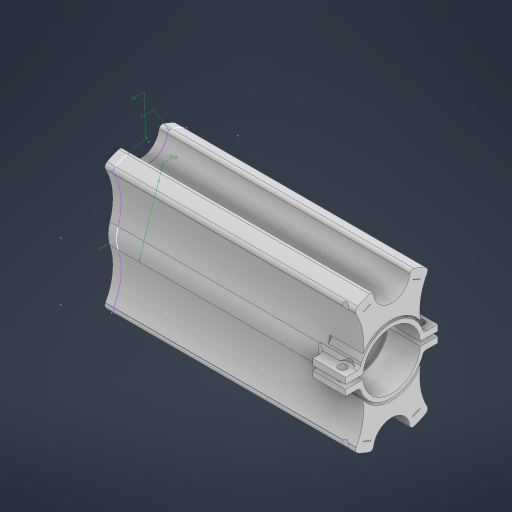
# Autodesk Inventor part: michigandrummy
Saved by Autodesk Inventor 2024.2 (Build 282272000, 272)
## iProperties
Created: 2024-04-03
Part Number: michigandrummy
Material: Generic
Document SubType Name: Modeling
Designer: jerem
Density: 1 g/cm^3
Appearance: Default
Author: jerem
## iProperties of the stored document michigandrummy_3DPrint.ipt
Created: 2024-04-05
Part Number: michigandrummy_3DPrint
Material: Generic
Document SubType Name: Modeling
Designer: jerem
Density: 1 g/cm^3
Appearance: Default
Author: jerem
Autodesk Inventor part; units mm, degrees
ref_plane "YZ Plane" through (0, 0, 0) normal (1, 0, 0) x (0, 1, 0)
ref_plane "XZ Plane" through (0, 0, 0) normal (0, 1, 0) x (-1, 0, 0)
ref_plane "XY Plane" through (0, 0, 0) normal (0, 0, 1) x (1, 0, 0)
sketch "Sketch1" plane through (0, 0, 0) normal (1, 0, 0) x (0, 1, 0)
  arc A0 (1, -13.863982) -> (1, 13.863982) centre (0, 0) ccw
  line L0 (0, 0) -> (1, 0) construction
  line L1 (1, 13.863982) -> (1, 22.388632)
  line L2 (1, 22.388632) -> (4, 22.388632)
  line L3 (4, 22.388632) -> (4, 15.388632)
  line L4 (1, -13.863982) -> (1, -22.388632)
  line L5 (1, -22.388632) -> (4, -22.388632)
  line L6 (4, -22.388632) -> (4, -15.388632)
  arc A1 (4, -15.388632) -> (4, 15.388632) centre (0, 0) ccw
  point P0 (4, -15.388632)
  point P1 (4, 15.388632)
  dimension "d0" = 27.8
  dimension "d1" = 1
  dimension "d3" = 3
  dimension "d4" = 2
  dimension "d5" = 1
  dimension "d11" = 7
  constraints: 14 end point, 4 point on circle, 2 centre point, 2 coincident, 2 collinear, 2 horizontal, 2 symmetric about line, 1 perpendicular, 1 vertical
  measures "d0" diameter of A0
  measures "d1" distance of L0.start L0.end
  measures "d3" distance of L1.end L2.end
  measures "d4" radial gap between concentric circles of A0 A1
  measures "d5" distance from line of point (0, 0) L1
  measures "d11" distance of L3.end L2.end
extrude "Extrusion1" add sketch "Sketch1" along normal blind 16
sketch "Sketch2" plane through (0, 4, 22.388632) normal (0, 1, 0) x (1, 0, 0)
  line L0 (0, 7) -> (16, 7) construction
  line L1 (16, 0) -> (16, 8.52465) construction
  line L2 (16, 7) -> (16, 0) construction
  circle A0 centre (11, 3.5) radius 2
  line L3 (16, 36.252614) -> (16, 8.52465)
  line L4 (16, 22.388632) -> (0, 22.388632)
  circle A1 centre (11, 41.277264) radius 2
  line L5 (11, 41.277264) -> (11, 37.777264) construction
  line L6 (0, 37.777264) -> (16, 37.777264) construction
  line L7 (11, 3.5) -> (11, 7) construction
  point P0 (16, 3.5)
  dimension "d8" = 5
  dimension "d9" = 4
  dimension "d10" = 3.5
  constraints: 8 end point, 3 point on line, 2 centre point, 2 midpoint, 1 collinear, 1 horizontal, 1 symmetric about line, 1 vertical, 1 other
  measures "d8" distance of point (16, 3.5) L7.start
  measures "d9" diameter of A0
  measures "d10" distance of L7.start L7.end
extrude "Extrusion2" cut sketch "Sketch2" along normal through all both and the other way through all
mirror "Mirror1" about plane through (0, 0, 0) normal (0, 1, 0) of "Extrusion1", "Extrusion2"
fillet "Fillet1" radius 2 4 edges at (8, 4, 15.3886) (8, -4, 15.3886) (8, 4, -15.3886) (8, -4, -15.3886)
sketch "Sketch3" plane through (0, -4, -22.388632) normal (-1, 0, 0) x (0, 0, 1)
  circle A0 centre (22.388632, 4) radius 13.9
  circle A1 centre (22.388632, 4) radius 15.9
  circle A2 centre (22.388632, 4) radius 4.85
  dimension "d15" = 9.7
  dimension "d19" = 27.8
  dimension "d20" = 2
  constraints: 3 centre point, 3 coincident
  measures "d15" diameter of A2
  measures "d19" diameter of A0
  measures "d20" radial gap between concentric circles of A0 A1
extrude "Extrusion3" add sketch "Sketch3" along normal blind 4.2 contours A0 | A1
sketch "Sketch4" plane through (-4.2, 0, 0) normal (-1, 0, 0) x (0, 0, 1)
  circle A0 centre (0, 0) radius 4.85 projected
  circle A1 centre (0, 0) radius 15.9
  circle A2 centre (0, 0) radius 4.85 projected
  circle A3 centre (0, 0) radius 1.8
  dimension "d18" = 3.6
  dimension "d21" = 31.8
  constraints: 2 centre point, 2 coincident
  measures "d18" diameter of A3
  measures "d21" diameter of A1
extrude "Extrusion4" add sketch "Sketch4" along normal blind 10 contours A0 | A1
fillet "Fillet2" radius 4 4 edges at (0, -3.1958, 15.5755) (0, 3.1958, 15.5755) (0, -3.1958, -15.5755) (0, 3.1958, -15.5755)
sketch "Sketch5" plane through (-14.2, 0, 0) normal (-1, 0, 0) x (0, 0, 1)
  circle A0 centre (0, 0) radius 1.8 projected
  circle A1 centre (0, 0) radius 2
  circle A2 centre (0, 0) radius 4
  dimension "d25" = 4
  dimension "d26" = 2
  constraints: 2 centre point, 2 coincident
  measures "d25" diameter of A1
  measures "d26" radial gap between concentric circles of A1 A2
extrude "Extrusion5" add sketch "Sketch5" along normal blind 87.8 contours A2
sketch "Sketch6" plane through (0, 0, 0) normal (1, 0, 0) x (0, 1, 0)
  circle A0 centre (0, 0) radius 1.8 construction
  circle A1 centre (0, 0) radius 35 construction
  line L0 (35, 0) -> (25, 0)
  line L1 (31.653557, -14.934936) -> (22.609684, -10.667811)
  arc A2 (31.653557, -14.934936) -> (35, 0) centre (0, 0) ccw construction
  dimension "d29" = 70
  dimension "d30" = 10
  dimension "d31" = 10
  constraints: 4 end point, 4 point on circle, 2 centre point, 1 coincident, 1 concentric, 1 horizontal, 1 line through centre
  measures "d29" diameter of A1
  measures "d30" distance of L0.start L0.end
  measures "d31" distance of L1.start L1.end
sketch "Sketch7" plane through (-102, 0, 0) normal (-1, 0, 0) x (0, 0, 1)
  circle A0 centre (0, 0) radius 15.9
  circle A1 centre (0, 0) radius 1.8
  line L0 (0, 0) -> (24.747716, 0) construction
  line L1 (-24.908169, 0) -> (-15.9, 0)
  line L2 (-1.8, 0) -> (15.9, 0)
  line L3 (17.349325, 28.247602) -> (17.271273, 28.112413)
  line L4 (0.160452, 0) -> (15.9, 0)
  arc A2 (0, 24.132295) -> (8.826003, 31.826928) centre (0, 33.041473) ccw
  arc A3 (17.349325, 28.247602) -> (15.118967, 4.922077) centre (43.063145, 14.019484) ccw
  arc A4 (0, 24.132295) -> (8.851951, 32.033302) centre (0, 33.041473) ccw
  arc A5 (16.480993, 30.876801) -> (10.805405, 33.290287) centre (0, 0) ccw
  line L5 (0, 15.9) -> (0, 24.132295)
  line L6 (-17.349325, 28.247602) -> (-17.271273, 28.112413)
  arc A6 (-15.118967, 4.922077) -> (-17.349325, 28.247602) centre (-43.063145, 14.019484) ccw
  arc A7 (-8.851951, 32.033302) -> (0, 24.132295) centre (0, 33.041473) ccw
  arc A8 (-10.805405, 33.290287) -> (-16.480993, 30.876801) centre (0, 0) ccw
  arc A9 (-16.480993, 30.876801) -> (-17.271273, 28.112413) centre (-15.539222, 29.112413) ccw
  arc A10 (17.271273, 28.112413) -> (16.480993, 30.876801) centre (15.539222, 29.112413) ccw
  arc A11 (-8.851951, 32.033302) -> (-10.805405, 33.290287) centre (-10.342316, 31.863561) ccw
  arc A12 (10.805405, 33.290287) -> (8.851951, 32.033302) centre (10.342316, 31.863561) ccw
  line L7 (17.349325, -28.247602) -> (17.271273, -28.112413)
  arc A13 (8.826003, -31.826928) -> (0, -24.132295) centre (0, -33.041473) ccw
  arc A14 (15.118967, -4.922077) -> (17.349325, -28.247602) centre (43.063145, -14.019484) ccw
  arc A15 (8.851951, -32.033302) -> (0, -24.132295) centre (0, -33.041473) ccw
  arc A16 (10.805405, -33.290287) -> (16.480993, -30.876801) centre (0, 0) ccw
  line L8 (0, -15.9) -> (0, -24.132295)
  arc A17 (-16.480993, -30.876801) -> (-10.805405, -33.290287) centre (0, 0) ccw
  arc A18 (-17.349325, -28.247602) -> (-15.118967, -4.922077) centre (-43.063145, -14.019484) ccw
  line L9 (-17.349325, -28.247602) -> (-17.271273, -28.112413)
  arc A19 (0, -24.132295) -> (-8.851951, -32.033302) centre (0, -33.041473) ccw
  arc A20 (-17.271273, -28.112413) -> (-16.480993, -30.876801) centre (-15.539222, -29.112413) ccw
  arc A21 (16.480993, -30.876801) -> (17.271273, -28.112413) centre (15.539222, -29.112413) ccw
  arc A22 (-10.805405, -33.290287) -> (-8.851951, -32.033302) centre (-10.342316, -31.863561) ccw
  arc A23 (8.851951, -32.033302) -> (10.805405, -33.290287) centre (10.342316, -31.863561) ccw
  point P0 (18.274622, 29.850263)
  point P1 (-8.826003, 31.826928)
  point P2 (-18.274622, 29.850263)
  point P3 (18.274622, -29.850263)
  point P4 (-8.826003, -31.826928)
  point P5 (-18.274622, -29.850263)
  point P6 (8.826003, 31.826928)
  point P7 (-15.118967, 4.922077)
  point P8 (-15.118967, -4.922077)
  point P9 (15.118967, -4.922077)
  dimension "d36" = 35
  dimension "d40" = 1.5
  dimension "d41" = 31.8
  constraints: 54 point on circle, 30 symmetric about line, 23 centre point, 20 end point, 9 tangent, 6 point on line, 4 coincident, 2 equal radius, 1 horizontal, 1 horizontal alignment, 15 other
  measures "d36" radius of A5
  measures "d40" radius of A11
  measures "d41" diameter of A0
extrude "Extrusion6" add sketch "Sketch7" against normal up to surface (87.8 mm away)
sketch "Sketch8" plane through (-14.2, 0, 0) normal (1, 0, 0) x (0, 0, -1)
  circle A0 centre (0, 0) radius 35
  circle A1 centre (0, 0) radius 15.9
  arc A2 (-17.349325, -28.247602) -> (-15.118967, -4.922077) centre (-43.063145, -14.019484) ccw
  arc A3 (15.118967, 4.922077) -> (-15.118967, 4.922077) centre (0, 0) ccw
  arc A4 (17.349325, 28.247602) -> (15.118967, 4.922077) centre (43.063145, 14.019484) ccw
  line L0 (17.349325, 28.247602) -> (17.271273, 28.112413)
  arc A5 (17.271273, 28.112413) -> (16.480993, 30.876801) centre (15.539222, 29.112413) ccw
  arc A6 (16.480993, 30.876801) -> (10.805405, 33.290287) centre (0, 0) ccw
  arc A7 (10.805405, 33.290287) -> (8.851951, 32.033302) centre (10.342316, 31.863561) ccw
  arc A8 (-8.851951, 32.033302) -> (8.851951, 32.033302) centre (0, 33.041473) ccw
  arc A9 (-8.851951, 32.033302) -> (-10.805405, 33.290287) centre (-10.342316, 31.863561) ccw
  arc A10 (-10.805405, 33.290287) -> (-16.480993, 30.876801) centre (0, 0) ccw
  arc A11 (-16.480993, 30.876801) -> (-17.271273, 28.112413) centre (-15.539222, 29.112413) ccw
  line L1 (-17.271273, 28.112413) -> (-17.349325, 28.247602)
  arc A12 (-15.118967, 4.922077) -> (-17.349325, 28.247602) centre (-43.063145, 14.019484) ccw
  arc A13 (-15.118967, -4.922077) -> (15.118967, -4.922077) centre (0, 0) ccw
  arc A14 (-17.349325, -28.247602) -> (-15.118967, -4.922077) centre (-43.063145, -14.019484) ccw
  line L2 (-17.349325, -28.247602) -> (-17.271273, -28.112413)
  arc A15 (-17.271273, -28.112413) -> (-16.480993, -30.876801) centre (-15.539222, -29.112413) ccw
  arc A16 (-16.480993, -30.876801) -> (-10.805405, -33.290287) centre (0, 0) ccw
  arc A17 (-10.805405, -33.290287) -> (-8.851951, -32.033302) centre (-10.342316, -31.863561) ccw
  arc A18 (8.851951, -32.033302) -> (-8.851951, -32.033302) centre (0, -33.041473) ccw
  arc A19 (8.851951, -32.033302) -> (10.805405, -33.290287) centre (10.342316, -31.863561) ccw
  arc A20 (10.805405, -33.290287) -> (16.480993, -30.876801) centre (0, 0) ccw
  arc A21 (16.480993, -30.876801) -> (17.271273, -28.112413) centre (15.539222, -29.112413) ccw
  line L3 (17.271273, -28.112413) -> (17.349325, -28.247602)
  arc A22 (15.118967, -4.922077) -> (17.349325, -28.247602) centre (43.063145, -14.019484) ccw
  point P0 (16.480993, 30.876801)
  point P1 (10.805405, 33.290287)
  point P2 (-10.805405, 33.290287)
  point P3 (-16.480993, 30.876801)
  point P4 (15.118967, 4.922077)
  point P5 (-17.349325, -28.247602)
  point P6 (-16.480993, -30.876801)
  point P7 (-10.805405, -33.290287)
  point P8 (10.805405, -33.290287)
  point P9 (16.480993, -30.876801)
  point P10 (15.118967, -4.922077)
  dimension "d44" = 70
  constraints: 2 coincident, 1 centre point, 2 other
  measures "d44" diameter of A0
extrude "Extrusion7" add sketch "Sketch8" along normal up to surface (30.2 mm away) contours A5 L0 A4 A1 A12 L1 A11 A0 A9 A8 A7 | A0 A19 A18 A17 A15 L2 A2 A1 A22 L3 A21
sketch "Sketch10" plane through (0, 4, 22.388632) normal (0, 1, 0) x (1, 0, 0)
  circle A0 centre (11, 3.5) radius 2
  circle A1 centre (11, 41.277264) radius 2
  circle A2 centre (11, 3.5) radius 2
  circle A3 centre (11, 41.277264) radius 2
  point P0 (0, 22.388632)
  point P1 (12.818889, 5.524172)
  point P2 (9.383152, 5.524172)
  point P3 (9.383152, 39.253092)
  point P4 (12.818889, 39.253092)
  point P5 (9.751783, 39.714589)
  point P6 (12.336765, 39.789629)
  point P7 (12.336765, 4.987635)
  point P8 (9.751783, 5.062675)
  constraints: 2 centre point, 2 coincident, 4 other
extrude "Extrusion8" cut sketch "Sketch10" along normal mid plane 147.627
sketch "Sketch12" plane through (16, 0, 0) normal (1, 0, 0) x (0, 0, -1)
  arc A0 (17.349325, 28.247602) -> (15.026237, 5.212004) centre (43.063145, 14.019484) ccw
  line L0 (17.271273, 28.112413) -> (17.349325, 28.247602)
  arc A1 (17.271273, 28.112413) -> (16.480993, 30.876801) centre (15.539222, 29.112413) ccw
  arc A2 (16.480993, 30.876801) -> (10.805405, 33.290287) centre (0, 0) ccw
  arc A3 (10.805405, 33.290287) -> (8.851951, 32.033302) centre (10.342316, 31.863561) ccw
  arc A4 (-8.851951, 32.033302) -> (8.851951, 32.033302) centre (0, 33.041473) ccw
  arc A5 (-8.851951, 32.033302) -> (-10.805405, 33.290287) centre (-10.342316, 31.863561) ccw
  arc A6 (-10.805405, 33.290287) -> (-16.480993, 30.876801) centre (0, 0) ccw
  arc A7 (-16.480993, 30.876801) -> (-17.271273, 28.112413) centre (-15.539222, 29.112413) ccw
  line L1 (-17.349325, 28.247602) -> (-17.271273, 28.112413)
  arc A8 (-15.026237, 5.212004) -> (-17.349325, 28.247602) centre (-43.063145, 14.019484) ccw
  arc A9 (-16.86446, 4) -> (-15.026237, 5.212004) centre (-16.86446, 6) ccw
  line L2 (-16.86446, 4) -> (-22.388632, 4)
  line L3 (-22.388632, 4) -> (-22.388632, 1)
  line L4 (-22.388632, 1) -> (-13.863982, 1)
  arc A10 (13.863982, 1) -> (-13.863982, 1) centre (0, 0) ccw
  line L5 (13.863982, 1) -> (22.388632, 1)
  line L6 (22.388632, 1) -> (22.388632, 4)
  line L7 (22.388632, 4) -> (16.86446, 4)
  arc A11 (15.026237, 5.212004) -> (16.86446, 4) centre (16.86446, 6) ccw
  line L8 (-13.933156, 27.332668) -> (-10.275527, 28.883084)
  line L9 (-10.275527, 28.883084) -> (-10.197472, 28.698944)
  line L10 (-10.197472, 28.698944) -> (-13.855102, 27.148528)
  line L11 (-13.855102, 27.148528) -> (-13.933156, 27.332668)
  line L12 (-14.20925, 31.985891) -> (-14.20925, 31.985891)
  point P0 (-17.310299, 28.180007)
  point P1 (-13.894129, 27.240598)
  point P2 (-10.236499, 28.791014)
  point P3 (-12.104342, 28.107876)
  dimension "d63" = 0.2
  constraints: 10 end point, 4 midpoint, 3 perpendicular, 2 point on circle, 1 tangent
  measures "d63" distance from line of L10 point (-12.104, 28.108)
extrude "Extrusion10" cut sketch "Sketch12" against normal through all contours L8 L9 L10 L11
mirror "Mirror4" about plane through (0, 0, 0) normal (0, 1, 0) of "Extrusion10"
mirror "Mirror5" about plane through (0, 0, 0) normal (0, 0, 1) of "Extrusion10", "Mirror4"
extrude "Extrusion12" add sketch "Sketch7" along normal blind 4
sketch "Sketch13" plane through (-102, 0, 0) normal (-1, 0, 0) x (0, 0, 1)
  circle A0 centre (0, 0) radius 3.925
  circle A1 centre (0, 0) radius 1.8 projected
  circle A2 centre (0, 0) radius 2
  dimension "d64" = 7.85
  dimension "d65" = 4
  constraints: 2 centre point, 2 coincident
  measures "d64" diameter of A0
  measures "d65" diameter of A2
extrude "Extrusion11" add sketch "Sketch13" along normal blind 10 from surface at 4 contours A0
sketch "Sketch14" plane through (-106, 0, 0) normal (-1, 0, 0) x (0, 0, 1)
  circle A0 centre (0, 0) radius 4.445
  circle A1 centre (0, 0) radius 2
  dimension "d70" = 8.89
  constraints: 2 centre point, 2 coincident
  measures "d70" diameter of A0
extrude "Extrusion13" add sketch "Sketch14" along normal blind 2 contours A0 | A1
sketch "Sketch15" plane through (16, 0, 0) normal (1, 0, 0) x (0, 0, -1)
  circle A0 centre (0, 0) radius 14
  dimension "d73" = 28
  constraints: 1 centre point, 1 coincident
  measures "d73" diameter of A0
extrude "Extrusion14" cut sketch "Sketch15" against normal up to surface (16 mm away)
sketch "Sketch16" plane through (0, 4, 22.388632) normal (0, 1, 0) x (1, 0, 0)
  circle A0 centre (11, 3.5) radius 2 projected
  circle A1 centre (11, 3.5) radius 4
  point P0 (0, 22.388632)
  dimension "d76" = 8
  constraints: 1 centre point, 1 coincident
  measures "d76" diameter of A1
extrude "Extrusion15" cut sketch "Sketch16" along normal blind 10
mirror "Mirror6" about plane through (0, 0, 0) normal (0, 1, 0) of "Extrusion15"
mirror "Mirror7" about plane through (0, 0, 0) normal (0, 0, 1) of "Extrusion15", "Mirror6"
sketch "Sketch17" plane through (16, 0, 0) normal (1, 0, 0) x (0, 0, -1)
  circle A0 centre (0, 0) radius 4.85
  circle A1 centre (0, 0) radius 16
  circle A2 centre (0, 0) radius 1.8
  circle A3 centre (0, 0) radius 17
  arc A4 (13.96424, 1) -> (-13.96424, 1) centre (0, 0) ccw
  line L0 (13.96424, 1) -> (22.388632, 1)
  line L1 (22.388632, 1) -> (22.388632, 4)
  line L2 (22.388632, 4) -> (16.86446, 4)
  arc A5 (15.026237, 5.212004) -> (16.86446, 4) centre (16.86446, 6) ccw
  arc A6 (17.349325, 28.247602) -> (15.026237, 5.212004) centre (43.063145, 14.019484) ccw
  line L3 (17.271273, 28.112413) -> (17.349325, 28.247602)
  arc A7 (17.271273, 28.112413) -> (16.480993, 30.876801) centre (15.539222, 29.112413) ccw
  arc A8 (16.480993, 30.876801) -> (10.805405, 33.290287) centre (0, 0) ccw
  arc A9 (10.805405, 33.290287) -> (8.851951, 32.033302) centre (10.342316, 31.863561) ccw
  arc A10 (-8.851951, 32.033302) -> (8.851951, 32.033302) centre (0, 33.041473) ccw
  arc A11 (-8.851951, 32.033302) -> (-10.805405, 33.290287) centre (-10.342316, 31.863561) ccw
  arc A12 (-10.805405, 33.290287) -> (-16.480993, 30.876801) centre (0, 0) ccw
  arc A13 (-16.480993, 30.876801) -> (-17.271273, 28.112413) centre (-15.539222, 29.112413) ccw
  line L4 (-17.349325, 28.247602) -> (-17.271273, 28.112413)
  arc A14 (-15.026237, 5.212004) -> (-17.349325, 28.247602) centre (-43.063145, 14.019484) ccw
  arc A15 (-16.86446, 4) -> (-15.026237, 5.212004) centre (-16.86446, 6) ccw
  line L5 (-16.86446, 4) -> (-22.388632, 4)
  line L6 (-22.388632, 4) -> (-22.388632, 1)
  line L7 (-22.388632, 1) -> (-13.96424, 1)
  line L8 (13.933156, 27.332668) -> (13.855102, 27.148528)
  line L9 (13.855102, 27.148528) -> (10.197472, 28.698944)
  line L10 (10.197472, 28.698944) -> (10.275527, 28.883084)
  line L11 (10.275527, 28.883084) -> (13.933156, 27.332668)
  line L12 (-10.275527, 28.883084) -> (-10.197472, 28.698944)
  line L13 (-10.197472, 28.698944) -> (-13.855102, 27.148528)
  line L14 (-13.855102, 27.148528) -> (-13.933156, 27.332668)
  line L15 (-13.933156, 27.332668) -> (-10.275527, 28.883084)
  arc A16 (-13.96424, -1) -> (13.96424, -1) centre (0, 0) ccw
  line L16 (-22.388632, -1) -> (-13.96424, -1)
  line L17 (-22.388632, -4) -> (-22.388632, -1)
  line L18 (-16.86446, -4) -> (-22.388632, -4)
  arc A17 (-15.026237, -5.212004) -> (-16.86446, -4) centre (-16.86446, -6) ccw
  arc A18 (-17.349325, -28.247602) -> (-15.026237, -5.212004) centre (-43.063145, -14.019484) ccw
  line L19 (-17.271273, -28.112413) -> (-17.349325, -28.247602)
  arc A19 (-17.271273, -28.112413) -> (-16.480993, -30.876801) centre (-15.539222, -29.112413) ccw
  arc A20 (-16.480993, -30.876801) -> (-10.805405, -33.290287) centre (0, 0) ccw
  arc A21 (-10.805405, -33.290287) -> (-8.851951, -32.033302) centre (-10.342316, -31.863561) ccw
  arc A22 (8.851951, -32.033302) -> (-8.851951, -32.033302) centre (0, -33.041473) ccw
  arc A23 (8.851951, -32.033302) -> (10.805405, -33.290287) centre (10.342316, -31.863561) ccw
  arc A24 (10.805405, -33.290287) -> (16.480993, -30.876801) centre (0, 0) ccw
  arc A25 (16.480993, -30.876801) -> (17.271273, -28.112413) centre (15.539222, -29.112413) ccw
  line L20 (17.349325, -28.247602) -> (17.271273, -28.112413)
  arc A26 (15.026237, -5.212004) -> (17.349325, -28.247602) centre (43.063145, -14.019484) ccw
  arc A27 (16.86446, -4) -> (15.026237, -5.212004) centre (16.86446, -6) ccw
  line L21 (22.388632, -4) -> (16.86446, -4)
  line L22 (22.388632, -1) -> (22.388632, -4)
  line L23 (13.96424, -1) -> (22.388632, -1)
  line L24 (-13.933156, -27.332668) -> (-13.855102, -27.148528)
  line L25 (-13.855102, -27.148528) -> (-10.197472, -28.698944)
  line L26 (-10.197472, -28.698944) -> (-10.275527, -28.883084)
  line L27 (-10.275527, -28.883084) -> (-13.933156, -27.332668)
  line L28 (13.855102, -27.148528) -> (13.933156, -27.332668)
  line L29 (13.933156, -27.332668) -> (10.275527, -28.883084)
  line L30 (10.275527, -28.883084) -> (10.197472, -28.698944)
  line L31 (10.197472, -28.698944) -> (13.855102, -27.148528)
  point P0 (14.003841, -9.638072)
  point P1 (14.707201, -6.300655)
  point P2 (-14.707201, -6.300655)
  point P3 (-14.003841, -9.638072)
  point P4 (-14.003841, 9.638072)
  point P5 (-14.707201, 6.300655)
  point P6 (14.707201, 6.300655)
  point P7 (14.003841, 9.638072)
  dimension "d79" = 32
  dimension "d80" = 34
  constraints: 2 centre point, 2 coincident
  measures "d79" diameter of A1
  measures "d80" diameter of A3
extrude "Extrusion16" cut sketch "Sketch17" against normal up to surface (16 mm away) contours A1 A14 A3 A6 | A26 A3 A18 A1
sketch "Sketch11" plane through (16, 0, 0) normal (1, 0, 0) x (0, 0, -1)
  line L0 (-15.513967, 28.277718) -> (-16.383128, 27.783189)
  line L1 (-16.383128, 27.783189) -> (-16.813972, 29.551486)
  line L2 (-16.813972, 29.551486) -> (-15.513967, 28.277718)
  arc A0 (17.349325, 28.247602) -> (15.026237, 5.212004) centre (43.063145, 14.019484) ccw
  line L3 (17.271273, 28.112413) -> (17.349325, 28.247602)
  arc A1 (17.271273, 28.112413) -> (16.480993, 30.876801) centre (15.539222, 29.112413) ccw
  arc A2 (16.480993, 30.876801) -> (10.805405, 33.290287) centre (0, 0) ccw
  arc A3 (10.805405, 33.290287) -> (8.851951, 32.033302) centre (10.342316, 31.863561) ccw
  arc A4 (-8.851951, 32.033302) -> (8.851951, 32.033302) centre (0, 33.041473) ccw
  arc A5 (-8.851951, 32.033302) -> (-10.805405, 33.290287) centre (-10.342316, 31.863561) ccw
  arc A6 (-10.805405, 33.290287) -> (-16.480993, 30.876801) centre (0, 0) ccw
  arc A7 (-16.480993, 30.876801) -> (-17.271273, 28.112413) centre (-15.539222, 29.112413) ccw
  line L4 (-17.349325, 28.247602) -> (-17.271273, 28.112413)
  arc A8 (-15.026237, 5.212004) -> (-17.349325, 28.247602) centre (-43.063145, 14.019484) ccw
  arc A9 (-16.86446, 4) -> (-15.026237, 5.212004) centre (-16.86446, 6) ccw
  line L5 (-16.86446, 4) -> (-20.388632, 4)
  line L6 (-20.388632, 4) -> (-20.388632, 1)
  line L7 (-20.388632, 1) -> (-13.863982, 1)
  arc A10 (13.863982, 1) -> (-13.863982, 1) centre (0, 0) ccw
  line L8 (13.863982, 1) -> (20.388632, 1)
  line L9 (20.388632, 1) -> (20.388632, 4)
  line L10 (20.388632, 4) -> (16.86446, 4)
  arc A11 (15.026237, 5.212004) -> (16.86446, 4) centre (16.86446, 6) ccw
  circle A12 centre (0, 0) radius 1.8 construction
  circle A13 centre (0, 0) radius 35 construction
  line L11 (-16.813972, 29.551486) -> (-15.948547, 28.030454) construction
  line L12 (-15.244324, 30.390962) -> (-14.45969, 28.826721) construction
  line L13 (-14.906616, 28.60254) -> (-15.244324, 30.390962)
  line L14 (-15.244324, 30.390962) -> (-14.012764, 29.050903)
  line L15 (-14.012764, 29.050903) -> (-14.906616, 28.60254)
  line L16 (-13.632892, 31.147139) -> (-12.931199, 29.543977) construction
  line L17 (-13.389246, 29.343493) -> (-13.632892, 31.147139)
  line L18 (-13.632892, 31.147139) -> (-12.473153, 29.744461)
  line L19 (-12.473153, 29.744461) -> (-13.389246, 29.343493)
  line L20 (-11.984094, 31.817943) -> (-11.367265, 30.180255) construction
  line L21 (-11.835176, 30.004018) -> (-11.984094, 31.817943)
  line L22 (-11.984094, 31.817943) -> (-10.899354, 30.356491)
  line L23 (-10.899354, 30.356491) -> (-11.835176, 30.004018)
  line L24 (-10.302447, 32.401537) -> (-9.772174, 30.733811) construction
  line L25 (-10.248668, 30.582304) -> (-10.302447, 32.401537)
  line L26 (-10.302447, 32.401537) -> (-9.295681, 30.885317)
  line L27 (-9.295681, 30.885317) -> (-10.248668, 30.582304)
  line L28 (-16.383128, 27.783189) -> (-16.94594, 27.492846) construction
  line L29 (-9.295681, 30.885317) -> (-8.678769, 31.028411) construction
  arc A14 (-8.851951, 32.033302) -> (8.851951, 32.033302) centre (0, 33.041473) ccw construction
  dimension "d49" = 34
  dimension "d50" = 1.75
  dimension "d51" = 1
  dimension "d54" = 12
  constraints: 44 end point, 3 line through centre, 2 equal length, 2 point on circle, 1 centre point, 1 coincident, 1 concentric, 1 midpoint, 33 other
  measures "d49" distance of A13.centre L1.end
  measures "d50" distance of L1.end L11.end
  measures "d51" distance of L0.start L0.end
body "Solid1"
